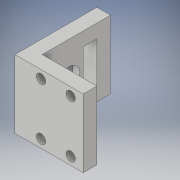
# Autodesk Inventor part: TensionerPlate
Saved by Autodesk Inventor 2017 (Build 210142000, 142)
## iProperties
Created: 2017-07-29
Part Number: TensionerPlate
Material: Generic
Document SubType Name: Modeling
Designer: User
Density: 1 g/cm^3
Appearance: Default
Author: User
Autodesk Inventor part; units mm, degrees
ref_plane "YZ Plane" through (0, 0, 0) normal (1, 0, 0) x (0, 1, 0)
ref_plane "XZ Plane" through (0, 0, 0) normal (0, 1, 0) x (-1, 0, 0)
ref_plane "XY Plane" through (0, 0, 0) normal (0, 0, 1) x (1, 0, 0)
sketch "Sketch4" plane through (0, 0, 0) normal (1, 0, 0) x (0, 1, 0)
  line L0 (0, 0) -> (31.75, 0)
  line L1 (31.75, 0) -> (31.75, -38.1)
  line L2 (31.75, -38.1) -> (0, -38.1)
  line L3 (0, -38.1) -> (0, 0)
  line L4 (25.4, -6.35) -> (6.35, -6.35)
  line L5 (6.35, -6.35) -> (6.35, -12.7)
  line L6 (6.35, -12.7) -> (25.4, -12.7)
  line L7 (25.4, -12.7) -> (25.4, -6.35)
  line L8 (25.4, -25.4) -> (6.35, -25.4)
  line L9 (6.35, -25.4) -> (6.35, -31.75)
  line L10 (6.35, -31.75) -> (25.4, -31.75)
  line L11 (25.4, -31.75) -> (25.4, -25.4)
  dimension "d36" = 31.75
  dimension "d37" = 38.1
  dimension "d38" = 19.05
  dimension "d39" = 6.35
  dimension "d40" = 6.35
  dimension "d41" = 6.35
  dimension "d42" = 6.35
  dimension "d43" = 6.35
  dimension "d44" = 6.35
  constraints: 24 end point, 6 parallel, 3 horizontal, 3 perpendicular
  measures "d36" distance of L1.end L2.end
  measures "d37" distance of L0.end L1.end
  measures "d38" distance of L6.end L5.end
  measures "d39" distance of L5.end L4.end
  measures "d40" distance between parallel lines of L4 L0
  measures "d41" distance between parallel lines of L1 L7
  measures "d42" distance of L8.end L9.end
  measures "d43" distance between parallel lines of L2 L10
  measures "d44" distance between parallel lines of L1 L11
extrude "Extrusion3" add sketch "Sketch4" along normal blind 6.35
sketch "Sketch5" plane through (6.35, 0, 0) normal (1, 0, 0) x (0, 0, -1)
  line L0 (25.4, 25.4) -> (31.75, 25.4) projected
  line L1 (31.75, 25.4) -> (31.75, 6.35) projected
  line L2 (31.75, 6.35) -> (25.4, 6.35) projected
  line L3 (25.4, 6.35) -> (25.4, 25.4) projected
  line L4 (6.35, 25.4) -> (12.7, 25.4) projected
  line L5 (12.7, 25.4) -> (12.7, 6.35) projected
  line L6 (12.7, 6.35) -> (6.35, 6.35) projected
  line L7 (6.35, 6.35) -> (6.35, 25.4) projected
  line L8 (0, 31.75) -> (0, 0) projected
  line L9 (0, 0) -> (38.1, 0) projected
  line L10 (38.1, 0) -> (38.1, 31.75) projected
  line L11 (38.1, 31.75) -> (0, 31.75) projected
  circle A0 centre (19.05, 15.875) radius 4.7625
  dimension "d47" = 9.525
  constraints: 1 centre point
  measures "d47" diameter of A0
extrude "Extrusion4" cut sketch "Sketch5" against normal blind 3.175 contours A0
sketch "Sketch6" plane through (0, 0, 0) normal (0, 0, 1) x (1, 0, 0)
  line L0 (3.175, 20.6375) -> (3.175, 11.1125) projected
  line L1 (0, 0) -> (0, 31.75) projected
  line L2 (0, 0) -> (6.35, 0) projected
  line L3 (6.35, 31.75) -> (6.35, 0) projected
  line L4 (0, 31.75) -> (6.35, 31.75) projected
  line L5 (0, 0) -> (6.35, 0) projected
  line L6 (0, 0) -> (31.75, 0)
  line L7 (31.75, 0) -> (31.75, 31.75)
  line L8 (31.75, 31.75) -> (0, 31.75)
  line L9 (0, 31.75) -> (0, 0)
  circle A0 centre (25.9588, 28.0162) radius 2.159
  circle A1 centre (25.9588, 3.7338) radius 2.159
  circle A2 centre (12.1412, 28.0162) radius 2.159
  circle A3 centre (12.1415, 3.8174) radius 2.159
  dimension "d50" = 31.75
  dimension "d51" = 4.318
  dimension "d53" = 3.7338
  dimension "d54" = 5.7912
  dimension "d55" = 4.318
  dimension "d56" = 4.318
  dimension "d57" = 4.318
  dimension "d58" = 13.8176
  dimension "d59" = 3.7338
  dimension "d60" = 13.8176
  dimension "d61" = 5.7912
  dimension "d64" = 3.7338
  constraints: 8 end point, 4 centre point, 2 parallel, 1 horizontal, 1 perpendicular
  measures "d50" distance of L8.end L7.end
  measures "d51" diameter of A0
  measures "d53" distance from line of L8 A0.centre
  measures "d54" distance from line of L7 A0.centre
  measures "d55" diameter of A1
  measures "d56" diameter of A2
  measures "d57" diameter of A3
  measures "d58" distance of A2.centre A0.centre
  measures "d59" distance from line of L8 A2.centre
  measures "d60" distance of A1.centre A3.centre
  measures "d61" distance from line of L7 A1.centre
  measures "d64" distance from line of L6 A1.centre
extrude "Extrusion5" add sketch "Sketch6" against normal blind 6.35 contours L3 L8 L7 L6
body "Solid2"
